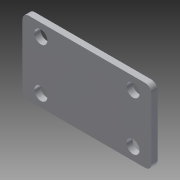
# Autodesk Inventor part: Aluminum Plate (0.125)
Saved by Autodesk Inventor 2014 (Build 180170000, 170)
## iProperties
Created: 2014-01-18
Part Number: Aluminum Plate (0.125)
Material: Aluminum 6061
Document SubType Name: Modeling
Designer: Andrew Toennies
Mass: 20.5908 g
Surface Area: 57.0457 cm^2
Volume: 7.59807 cm^3
Density: 2.71 g/cm^3
Appearance: Aluminum - Flat
Author: Andrew Toennies
Autodesk Inventor part; units mm, degrees
ref_plane "YZ Plane" through (0, 0, 0) normal (1, 0, 0) x (0, 1, 0)
ref_plane "XZ Plane" through (0, 0, 0) normal (0, 1, 0) x (-1, 0, 0)
ref_plane "XY Plane" through (0, 0, 0) normal (0, 0, 1) x (1, 0, 0)
sketch "Sketch1" plane through (0, 0, 0) normal (0, 0, 1) x (1, 0, 0)
  line L0 (3.175, 0) -> (63.627, 0)
  line L1 (66.802, 3.175) -> (66.802, 34.925)
  line L2 (63.627, 38.1) -> (3.175, 38.1)
  line L3 (0, 34.925) -> (0, 3.175)
  line L4 (9.525, 31.75) -> (57.277, 31.75) construction
  line L5 (57.277, 31.75) -> (57.277, 6.35) construction
  line L6 (57.277, 6.35) -> (9.525, 6.35) construction
  line L7 (9.525, 6.35) -> (9.525, 31.75) construction
  circle A0 centre (9.525, 31.75) radius 3.3782
  circle A1 centre (9.525, 6.35) radius 3.3782
  circle A2 centre (57.277, 31.75) radius 3.3782
  circle A3 centre (57.277, 6.35) radius 3.3782
  arc A4 (3.175, 38.1) -> (0, 34.925) centre (3.175, 34.925) ccw
  arc A5 (66.802, 34.925) -> (63.627, 38.1) centre (63.627, 34.925) ccw
  arc A6 (63.627, 0) -> (66.802, 3.175) centre (63.627, 3.175) ccw
  arc A7 (0, 3.175) -> (3.175, 0) centre (3.175, 3.175) ccw
  point P0 (0, 0)
  point P1 (66.802, 38.1)
  point P2 (0, 38.1)
  dimension "d0" = 38.1
  dimension "d1" = 66.802
  dimension "d2" = 25.4
  dimension "d3" = 47.752
  dimension "d4" = 9.525
  dimension "d5" = 6.35
  dimension "d6" = 6.7564
  dimension "d7" = 6.7564
  dimension "d8" = 6.7564
  dimension "d9" = 6.7564
  dimension "d10" = 3.175
  constraints: 16 end point, 8 centre point, 8 point on circle, 8 tangent, 6 point on line, 4 coincident, 4 parallel, 3 equal radius, 2 horizontal, 2 perpendicular
  measures "d0" distance of point (0, 38.1) point (0, 0)
  measures "d1" distance of point (66.802, 38.1) point (0, 38.1)
  measures "d2" distance of L6.end L4.start
  measures "d3" distance of L4.start L4.end
  measures "d4" distance between parallel lines of L1 L5
  measures "d5" distance between parallel lines of L2 L4
  measures "d6" diameter of A0
  measures "d7" diameter of A1
  measures "d8" diameter of A2
  measures "d9" diameter of A3
  measures "d10" radius of A4
extrude "Extrusion1" add sketch "Sketch1" along normal blind 3.175
equation "\"d4\" = -0.5 * d3 + 0.5 * d1"
equation "\"d5\" = -0.5 * d2 + 0.5 * d0"
body "Solid1"
